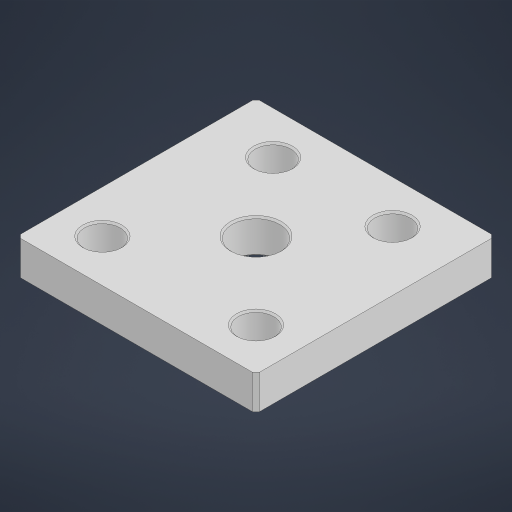
# Autodesk Inventor part: AP1-002
Saved by Autodesk Inventor 2024.3 (Build 283343000, 343)
## iProperties
Created: 2024-05-02
Part Number: AP1-002
Material: Generic
Document SubType Name: Modeling
Designer: fablabadmin
Density: 1 g/cm^3
Appearance: Default
Description: Plate top
Author: fablabadmin
Autodesk Inventor part; units mm, degrees
ref_plane "YZ Plane" through (0, 0, 0) normal (1, 0, 0) x (0, 1, 0)
ref_plane "XZ Plane" through (0, 0, 0) normal (0, 1, 0) x (-1, 0, 0)
ref_plane "XY Plane" through (0, 0, 0) normal (0, 0, 1) x (1, 0, 0)
sketch "Sketch1" plane through (0, 0, 0) normal (0, 1, 0) x (-1, 0, 0)
  line L0 (-35, 35) -> (35, 35)
  line L1 (35, 35) -> (35, -35)
  line L2 (35, -35) -> (-35, -35)
  line L3 (-35, -35) -> (-35, 35)
  line L4 (-35, 35) -> (35, -35) construction
  line L5 (35, 35) -> (-35, -35) construction
  line L6 (-22.5, 22.5) -> (22.5, 22.5) construction
  line L7 (22.5, 22.5) -> (22.5, -22.5) construction
  line L8 (22.5, -22.5) -> (-22.5, -22.5) construction
  line L9 (-22.5, -22.5) -> (-22.5, 22.5) construction
  line L10 (-22.5, 22.5) -> (22.5, -22.5) construction
  line L11 (22.5, 22.5) -> (-22.5, -22.5) construction
  line L12 (-17.5, 22.5) -> (17.5, 22.5) construction
  line L13 (17.5, 22.5) -> (17.5, -22.5) construction
  line L14 (17.5, -22.5) -> (-17.5, -22.5) construction
  line L15 (-17.5, -22.5) -> (-17.5, 22.5) construction
  line L16 (-17.5, 22.5) -> (17.5, -22.5) construction
  line L17 (17.5, 22.5) -> (-17.5, -22.5) construction
  circle A0 centre (0, 0) radius 7
  dimension "d0" = 70
  dimension "d1" = 45
  dimension "d2" = 35
  dimension "d3" = 14
  dimension "d16" = 70
  dimension "d17" = 45
  constraints: 36 end point, 6 midpoint, 6 parallel, 5 coincident, 5 perpendicular, 3 horizontal, 1 centre point, 1 point on line
  measures "d0" distance of L1.end L2.end
  measures "d1" distance of L7.end L8.end
  measures "d2" distance between parallel lines of L15 L13
  measures "d3" diameter of A0
  measures "d16" distance of L2.end L0.start
  measures "d17" distance of L8.end L6.start
extrude "Extrusion1" add sketch "Sketch1" against normal blind 10
hole "Hole1" at (-17.5, 0, -22.5) at (17.5, 0, -22.5) at (-22.5, 0, 22.5) at (22.5, 0, 22.5) direction (0, -1, 0) diameter 10.5 end through all
chamfer "Chamfer1" distance 0.5 angle 45 10 edges at (-17.5, 0, -27.75) (17.5, -10, -27.75) (17.5, 0, -27.75) (22.5, 0, 17.25) (22.5, -10, 17.25) (-22.5, 0, 17.25) (-22.5, -10, 17.25) (-17.5, -10, -27.75) (7, 0, 0) (7, -10, 0)
chamfer "Chamfer2" distance 1 angle 45 4 edges at (-35, -5, -35) (35, -5, -35) (35, -5, 35) (-35, -5, 35)
body "Solid1"
